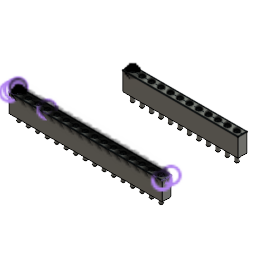
Penguin gameboy (Autodesk Fusion 360 archive; units mm, degrees)
design "Stacking headers 16/12 short v2"
Autodesk Fusion 360 part; units mm, degrees
note: some values were not read from the file. Chosen so that the rebuilt part matches the saved one: which bodies a step acts on.
sketch "Sketch1" plane through (0, 0, 0) normal (0, 1, 0) x (1, 0, 0)
  line L0 (0, 0) -> (41.04, 0)
  line L1 (41.04, 0) -> (41.04, -2.4)
  line L2 (41.04, -2.4) -> (0, -2.4)
  line L3 (0, -2.4) -> (0, 0)
  line L4 (41.04, -1.2) -> (0, -1.2) construction
  circle A0 centre (1.47, -1.2) radius 0.5
  circle A1 centre (4.01, -1.2) radius 0.5
  circle A2 centre (6.55, -1.2) radius 0.5
  circle A3 centre (9.09, -1.2) radius 0.5
  circle A4 centre (11.63, -1.2) radius 0.5
  circle A5 centre (14.17, -1.2) radius 0.5
  circle A6 centre (16.71, -1.2) radius 0.5
  circle A7 centre (19.25, -1.2) radius 0.5
  circle A8 centre (21.79, -1.2) radius 0.5
  circle A9 centre (24.33, -1.2) radius 0.5
  circle A10 centre (26.87, -1.2) radius 0.5
  circle A11 centre (29.41, -1.2) radius 0.5
  circle A12 centre (31.95, -1.2) radius 0.5
  circle A13 centre (34.49, -1.2) radius 0.5
  circle A14 centre (37.03, -1.2) radius 0.5
  circle A15 centre (39.57, -1.2) radius 0.5
  dimension "d1" = 41.04
  dimension "d2" = 2.4
  dimension "d3" = 1
  dimension "d4" = 1.47
  dimension "d11" = -38.1
  dimension "d12" = 0
  constraint horizontal L0
  constraint vertical L1
  constraint horizontal L2
  constraint vertical L3
  constraint coincident L0.start L3.end
  constraint midpoint L1 L4.start
  constraint midpoint L3 L4.end
  constraint coincident L4 A0.centre
  measures "d1" distance of L0.start L0.end
  measures "d2" distance of L0.start L2.end
  measures "d3" diameter of A0
  measures "d4" distance of L3 A0.centre
extrude "Extrude1" add sketch "Sketch1" against normal blind 7 contours A0 | A1 | A2 | A3 | A4 | A5 | A6 | A7 | A8 | A9 | A10 | A11 | A12 | A13 | A14 | A15 makes body 1 at (7.0475, -4.6667, 1.2498) makes body 2 at (16.3609, -4.6667, 0.8421) makes body 3 at (26.5209, -4.6667, 0.8421) makes body 4 at (36.8019, -2.3333, 1.6449) makes body 5 at (34.2619, -2.3333, 1.6449) makes body 6 at (23.9809, -4.6667, 0.8421) makes body 7 at (14.6675, -4.6667, 1.2498) makes body 8 at (4.5075, -4.6667, 1.2498) makes body 9 at (9.5875, -4.6667, 1.2498) makes body 10 at (18.9009, -4.6667, 0.8421) makes body 11 at (29.0609, -4.6667, 0.8421) makes body 12 at (39.3419, -2.3333, 1.6449) makes body 13 at (32.2213, -4.6667, 0.78) makes body 14 at (21.4409, -4.6667, 0.8421) makes body 15 at (12.1275, -4.6667, 1.2498) makes body 16 at (1.9675, -4.6667, 1.2498)
extrude "Extrude2" add sketch "Sketch1" against normal blind 5 bodies 1 2 3 4 5 6 7 8 9 10 11 12 13 14 15 16
fillet "Fillet1" radius 0.5 16 edges at (1.0038, -7, 1.0192) (3.5438, -7, 1.0192) (6.0838, -7, 1.0192) (8.6238, -7, 1.0192) (11.1638, -7, 1.0192) (13.7038, -7, 1.0192) (16.2438, -7, 1.0192) (18.7838, -7, 1.0192) (21.3238, -7, 1.0192) (23.8638, -7, 1.0192) (26.4038, -7, 1.0192) (28.9438, -7, 1.0192) (31.4838, -7, 1.0192) (34.0238, -7, 1.0192) (36.5638, -7, 1.0192) (39.1038, -7, 1.0192) on bodies 1
copy_body "Body->Comp1" bodies 1 removing the originals makes body 17 in component "Component"
sketch "Sketch1 (2)" plane through (0, 0, 0) normal (0, 1, 0) x (1, 0, 0) in component "Component"
  line L0 (10.16, 20.32) -> (41.04, 20.32)
  line L1 (41.04, 20.32) -> (41.04, 17.92)
  line L2 (41.04, 17.92) -> (10.16, 17.92)
  line L3 (10.16, 17.92) -> (10.16, 20.32)
  line L4 (41.04, 0) -> (41.04, -2.4)
  line L5 (41.04, 19.12) -> (10.16, 19.12) construction
  circle A0 centre (11.63, 19.12) radius 0.5
  circle A1 centre (14.17, 19.12) radius 0.5
  circle A2 centre (16.71, 19.12) radius 0.5
  circle A3 centre (19.25, 19.12) radius 0.5
  circle A4 centre (21.79, 19.12) radius 0.5
  circle A5 centre (24.33, 19.12) radius 0.5
  circle A6 centre (26.87, 19.12) radius 0.5
  circle A7 centre (29.41, 19.12) radius 0.5
  circle A8 centre (31.95, 19.12) radius 0.5
  circle A9 centre (34.49, 19.12) radius 0.5
  circle A10 centre (37.03, 19.12) radius 0.5
  circle A11 centre (39.57, 19.12) radius 0.5
  line L6 (0, -2.4) -> (0, 0)
  point P0 (9.09, -1.2)
  point P1 (0, -1.2)
  dimension "d19" = 30.88
  dimension "d20" = 2.4
  dimension "d21" = 1
  dimension "d22" = 1.47
  dimension "d25" = -27.94
  dimension "d26" = 0
  dimension "d27" = 20.32
  constraint horizontal L0
  constraint vertical L1
  constraint horizontal L2
  constraint vertical L3
  constraint midpoint L1 L5.start
  constraint midpoint L3 L5.end
  constraint coincident L5 A0.centre
  constraint collinear L1 L4
  measures "d19" distance of L0.start L0.end
  measures "d20" distance of L0.start L2.end
  measures "d21" diameter of A0
  measures "d22" distance of L3 A0.centre
  measures "d27" vertical distance of A0.centre P0
extrude "Extrude1'" add sketch "Sketch1 (2)" against normal blind 5 separate body makes body 18 in component "Component"
extrude "Extrude2'" add sketch "Sketch1 (2)" against normal blind 7.5 contours A11 bodies 18 in component "Component"
fillet "Fillet1'" radius 0.5 1 edges at (39.1038, -7.5, -19.3008) on bodies 18 in component "Component"
extrude "Extrude3" cut sketch "Sketch1 (2)" against normal blind 2.54 contours A11 bodies 18 in component "Component"
pattern_linear "R-Pattern1" count 12 spacing 2.54 along (-1, 0, 0) of "Extrude2'" in component "Component"
fillet "Fillet2" radius 0.5 11 edges at (36.5638, -7.5, -19.3008) (34.0238, -7.5, -19.3008) (31.4838, -7.5, -19.3008) (28.9438, -7.5, -19.3008) (26.4038, -7.5, -19.3008) (23.8638, -7.5, -19.3008) (21.3238, -7.5, -19.3008) (18.7838, -7.5, -19.3008) (16.2438, -7.5, -19.3008) (13.7038, -7.5, -19.3008) (11.1638, -7.5, -19.3008) on bodies 18 in component "Component"
extrude "Extrude4" cut sketch "Sketch1" against normal blind 2.54 contours A0 | A1 | A2 | A3 | A4 | A5 | A6 | A7 | A8 | A9 | A10 | A11 | A12 | A13 | A14 | A15 bodies 17 in component "Component"
extrude "Extrude5" cut sketch "Sketch1 (2)" against normal blind 4.5 contours A0 | A1 | A2 | A3 | A4 | A5 | A6 | A7 | A8 | A9 | A10 bodies 18 in component "Component"
component "Component" placed x (1, 0, 0) y (0, 1, 0) z (0, 0, 1) at (0, 0, 0)
equation "d1 = ( ( 2.54 * 16 ) * 1 mm ) + 0.4 mm"
equation "d11 = ( -2.54 * 15 ) * 1 mm"
equation "d19 = ( 2.54 * 12 ) * 1 mm + 0.4 mm"
equation "d25 = ( -2.54 * 11 ) * 1 mm"
equation "d38 = ( 2.54 * 11 ) * 1 mm"

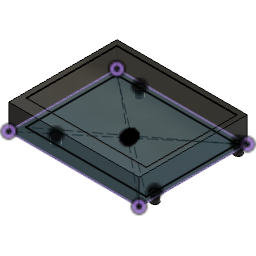
design "SCREEN"
part number: 2025-11-17-10-39-17-028
part number: 2025-11-20-10-21-56-898
Autodesk Fusion 360 part; units mm, degrees
sketch "Sketch1" plane through (0, 0, 0) normal (0, 1, 0) x (1, 0, 0) in component "screen"
  line L0 (38.3, 31.8) -> (-38.3, 31.8)
  line L1 (-38.3, 31.8) -> (-38.3, -31.8)
  line L2 (-38.3, -31.8) -> (38.3, -31.8)
  line L3 (38.3, -31.8) -> (38.3, 31.8)
  line L4 (38.3, 31.8) -> (-38.3, -31.8) construction
  line L5 (-38.3, 31.8) -> (38.3, -31.8) construction
  line L6 (35.34, 28.78) -> (-35.34, 28.78)
  line L7 (-35.34, 28.78) -> (-35.34, -24.58)
  line L8 (-35.34, -24.58) -> (35.34, -24.58)
  line L9 (35.34, -24.58) -> (35.34, 28.78)
  line L10 (35.34, 28.78) -> (-35.34, -24.58) construction
  line L11 (-35.34, 28.78) -> (35.34, -24.58) construction
  point P0 (0, 2.1)
  dimension "d1" = 63.6
  dimension "d2" = 76.6
  dimension "d3" = 70.68
  dimension "d4" = 53.36
  dimension "d7" = 2.96
  dimension "d8" = 3.02
  constraint horizontal L0
  constraint perpendicular L0 L1
  constraint parallel L0 L2
  constraint parallel L1 L3
  constraint coincident L4 origin
  constraint coincident L5 origin
  constraint horizontal L6
  constraint perpendicular L6 L7
  constraint parallel L6 L8
  constraint parallel L7 L9
  constraint coincident L10 P0
  constraint coincident L11 P0
  measures "d1" distance of L0.end L1.end
  measures "d2" distance of L0.start L0.end
  measures "d3" distance of L7.end L8.end
  measures "d4" distance of L6.end L7.end
  measures "d7" distance of L1 L7
  measures "d8" distance of L0 L6
extrude "Extrude1" add sketch "Sketch1" along normal blind 15 in component "screen"
extrude "Extrude2" add sketch "Sketch1" along normal blind 14.5 contours L6 L7 L8 L9 in component "screen"
sketch "Sketch2" plane through (0, 0, 0) normal (0, 1, 0) x (1, 0, 0) in component "screen"
  line L0 (-38.3, -31.8) -> (38.3, -31.8)
  circle A0 centre (35.29, -19.52) radius 2.32
  circle A1 centre (-22.71, -19.52) radius 2.32
  circle A2 centre (35.29, 29.48) radius 2.32
  circle A3 centre (-22.71, 29.48) radius 2.32
  line L1 (38.3, -31.8) -> (38.3, 31.8)
  line L2 (-38.3, 31.8) -> (-38.3, -31.8)
  line L3 (38.3, 31.8) -> (-38.3, 31.8)
  dimension "d17" = 12.28
  dimension "d20" = -58
  dimension "d21" = 49
  dimension "d24" = 15.59
  constraint tangent A2 L3
  measures "d17" distance of L0 A0.centre
  measures "d24" distance of A3.centre L2
extrude "Extrude3" add sketch "Sketch2" against normal blind 5 contours A2 | A3 | A0 | A1 in component "screen"
component "screen" placed x (1, 0, 0) y (0, 1, 0) z (0, 0, 1) at (0, 0, 0)
equation "d7 = ( 5.92 / 2 ) * 1 mm"

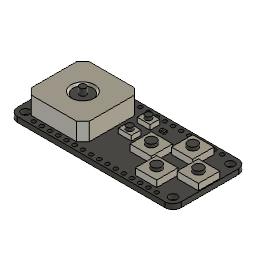
design "3632 Joy FeatherWing (bad)"
Autodesk Fusion 360 part; units mm, degrees
sketch "PCB" plane through (0, 0, 0) normal (0, 0, 1) x (1, 0, 0)
  arc A0 (50.8, 20.32) -> (48.26, 22.86) centre (48.26, 20.32) ccw
  arc A1 (48.26, 0) -> (50.8, 2.54) centre (48.26, 2.54) ccw
  line L0 (2.54, 22.86) -> (48.26, 22.86)
  line L1 (0, 20.32) -> (0, 2.54)
  circle A2 centre (5.43, 5.43) radius 0.8
  arc A3 (0, 2.54) -> (2.54, 0) centre (2.54, 2.54) ccw
  line L2 (48.26, 0) -> (2.54, 0)
  arc A4 (0, 2.54) -> (2.54, 0) centre (2.54, 2.54) ccw
  circle A5 centre (17.43, 17.43) radius 0.8
  arc A6 (50.8, 20.32) -> (48.26, 22.86) centre (48.26, 20.32) ccw
  line L3 (50.8, 2.54) -> (50.8, 20.32)
  arc A7 (48.26, 0) -> (50.8, 2.54) centre (48.26, 2.54) ccw
  line L4 (50.8, 20.32) -> (50.8, 2.54)
  line L5 (2.54, 0) -> (48.26, 0)
  arc A8 (2.54, 22.86) -> (0, 20.32) centre (2.54, 20.32) ccw
  arc A9 (2.54, 22.86) -> (0, 20.32) centre (2.54, 20.32) ccw
  line L6 (48.26, 22.86) -> (2.54, 22.86)
  line L7 (0, 2.54) -> (0, 20.32)
  circle A10 centre (2.54, 2.54) radius 1.27
  circle A11 centre (2.54, 20.32) radius 1.27
  circle A12 centre (2.43, 13.43) radius 0.635
  circle A13 centre (2.43, 11.43) radius 0.635
  circle A14 centre (2.43, 9.43) radius 0.635
  circle A15 centre (9.43, 20.43) radius 0.635
  circle A16 centre (11.43, 20.43) radius 0.635
  circle A17 centre (13.43, 20.43) radius 0.635
  circle A18 centre (48.26, 20.32) radius 1.27
  circle A19 centre (48.26, 2.54) radius 1.27
  circle A20 centre (6.35, 1.27) radius 0.635
  circle A21 centre (8.89, 1.27) radius 0.635
  circle A22 centre (11.43, 1.27) radius 0.635
  circle A23 centre (13.97, 1.27) radius 0.635
  circle A24 centre (16.51, 1.27) radius 0.635
  circle A25 centre (19.05, 1.27) radius 0.635
  circle A26 centre (21.59, 1.27) radius 0.635
  circle A27 centre (24.13, 1.27) radius 0.635
  circle A28 centre (26.67, 1.27) radius 0.635
  circle A29 centre (29.21, 1.27) radius 0.635
  circle A30 centre (31.75, 1.27) radius 0.635
  circle A31 centre (34.29, 1.27) radius 0.635
  circle A32 centre (36.83, 1.27) radius 0.635
  circle A33 centre (39.37, 1.27) radius 0.635
  circle A34 centre (41.91, 1.27) radius 0.635
  circle A35 centre (44.45, 1.27) radius 0.635
  circle A36 centre (16.51, 21.59) radius 0.635
  circle A37 centre (19.05, 21.59) radius 0.635
  circle A38 centre (21.59, 21.59) radius 0.635
  circle A39 centre (24.13, 21.59) radius 0.635
  circle A40 centre (26.67, 21.59) radius 0.635
  circle A41 centre (29.21, 21.59) radius 0.635
  circle A42 centre (31.75, 21.59) radius 0.635
  circle A43 centre (34.29, 21.59) radius 0.635
  circle A44 centre (36.83, 21.59) radius 0.635
  circle A45 centre (39.37, 21.59) radius 0.635
  circle A46 centre (41.91, 21.59) radius 0.635
  circle A47 centre (44.45, 21.59) radius 0.635
  dimension "d1" = 2.54
  dimension "d2" = 2.54
  dimension "d3" = 1.27
  dimension "d4" = 1.27
  dimension "d5" = 1.27
  dimension "d6" = 1.27
  dimension "d7" = 1.27
  dimension "d8" = 1.27
  dimension "d9" = 2.54
  dimension "d10" = 2.54
  dimension "d11" = 1.27
  dimension "d14" = 2.54
  dimension "d15" = 0
  dimension "d16" = 1.27
  dimension "d19" = 2.54
  dimension "d20" = 0
  constraint concentric A3 A10
  constraint concentric A8 A11
  constraint concentric A0 A18
  constraint concentric A1 A19
  measures "d1" diameter of A10
  measures "d2" diameter of A11
  measures "d3" diameter of A12
  measures "d4" diameter of A13
  measures "d5" diameter of A14
  measures "d6" diameter of A15
  measures "d7" diameter of A16
  measures "d8" diameter of A17
  measures "d9" diameter of A18
  measures "d10" diameter of A19
  measures "d11" diameter of A20
  measures "d16" diameter of A36
extrude "Extrude1" add sketch "PCB" along normal blind 1.6 makes body 1
sketch "thumbstick" plane through (0, 0, 1.6) normal (0, 0, 1) x (-1, 0, 0)
  circle A0 centre (-31.75, -21.59) radius 0.635
  circle A1 centre (-8.89, -1.27) radius 0.635
  circle A2 centre (-19.05, -1.27) radius 0.635
  circle A3 centre (-16.51, -1.27) radius 0.635
  circle A4 centre (-41.91, -21.59) radius 0.635
  circle A5 centre (-2.54, -2.54) radius 1.27 construction
  circle A6 centre (-39.37, -21.59) radius 0.635
  circle A7 centre (-24.13, -1.27) radius 0.635
  circle A8 centre (-13.97, -1.27) radius 0.635
  circle A9 centre (-36.83, -21.59) radius 0.635
  circle A10 centre (-48.26, -2.54) radius 1.27
  circle A11 centre (-6.35, -1.27) radius 0.635
  circle A12 centre (-11.43, -1.27) radius 0.635
  circle A13 centre (-2.43, -13.43) radius 0.635 construction
  circle A14 centre (-2.54, -20.32) radius 1.27 construction
  circle A15 centre (-44.45, -21.59) radius 0.635
  circle A16 centre (-17.43, -17.43) radius 0.8 construction
  circle A17 centre (-11.43, -20.43) radius 0.635 construction
  circle A18 centre (-9.43, -20.43) radius 0.635 construction
  circle A19 centre (-34.29, -1.27) radius 0.635
  circle A20 centre (-24.13, -21.59) radius 0.635
  circle A21 centre (-2.43, -9.43) radius 0.635 construction
  circle A22 centre (-31.75, -1.27) radius 0.635
  circle A23 centre (-2.43, -11.43) radius 0.635 construction
  circle A24 centre (-21.59, -1.27) radius 0.635
  circle A25 centre (-16.51, -21.59) radius 0.635
  circle A26 centre (-48.26, -20.32) radius 1.27
  circle A27 centre (-21.59, -21.59) radius 0.635
  circle A28 centre (-39.37, -1.27) radius 0.635
  circle A29 centre (-29.21, -1.27) radius 0.635
  circle A30 centre (-41.91, -1.27) radius 0.635
  circle A31 centre (-13.43, -20.43) radius 0.635 construction
  circle A32 centre (-34.29, -21.59) radius 0.635
  circle A33 centre (-26.67, -1.27) radius 0.635
  circle A34 centre (-26.67, -21.59) radius 0.635
  circle A35 centre (-19.05, -21.59) radius 0.635
  circle A36 centre (-44.45, -1.27) radius 0.635
  circle A37 centre (-36.83, -1.27) radius 0.635
  circle A38 centre (-29.21, -21.59) radius 0.635
  circle A39 centre (-5.43, -5.43) radius 0.8 construction
  line L0 (-2.54, 0) -> (-48.26, 0)
  arc A40 (-48.26, 0) -> (-50.8, -2.54) centre (-48.26, -2.54) ccw
  line L1 (-50.8, -2.54) -> (-50.8, -20.32)
  arc A41 (-50.8, -20.32) -> (-48.26, -22.86) centre (-48.26, -20.32) ccw
  line L2 (-48.26, -22.86) -> (-2.54, -22.86)
  arc A42 (-2.54, -22.86) -> (0, -20.32) centre (-2.54, -20.32) ccw
  line L3 (0, -20.32) -> (0, -2.54)
  arc A43 (0, -2.54) -> (-2.54, 0) centre (-2.54, -2.54) ccw
  line L4 (-20.43, -2.43) -> (-2.43, -2.43)
  line L5 (-2.43, -2.43) -> (-2.43, -20.43)
  line L6 (-2.43, -20.43) -> (-20.43, -20.43)
  line L7 (-20.43, -20.43) -> (-20.43, -2.43)
  line L8 (-20.43, -2.43) -> (-2.43, -20.43) construction
  line L9 (-2.43, -2.43) -> (-20.43, -20.43) construction
  point P0 (-11.43, -11.43)
  dimension "d23" = 18
  dimension "d24" = 18
  dimension "d25" = 11.43
  dimension "d26" = 11.43
  constraint perpendicular L4 L5
  constraint parallel L4 L6
  constraint parallel L5 L7
  constraint horizontal L4
  constraint coincident L8 P0
  constraint coincident L9 P0
  measures "d23" distance of L5.end L6.end
  measures "d24" distance of L4.end L5.end
  measures "d25" distance of L3 P0
  measures "d26" distance of L0 P0
extrude "Extrude2" add sketch "thumbstick" along normal blind 5.5 separate body contours L4 L5 L6 L7 makes body 2
chamfer "Chamfer1" distance 2 angle 45 4 edges at (2.43, 2.43, 4.35) (2.43, 20.43, 4.35) (20.43, 20.43, 4.35) (20.43, 2.43, 4.35) on bodies 2
sketch "stem" plane through (0, 0, 7.1) normal (0, 0, 1) x (-1, 0, 0)
  line L0 (-18.43, -2.43) -> (-20.43, -4.43)
  line L1 (-20.43, -4.43) -> (-20.43, -18.43)
  line L2 (-20.43, -18.43) -> (-18.43, -20.43)
  line L3 (-18.43, -20.43) -> (-4.43, -20.43)
  line L4 (-4.43, -20.43) -> (-2.43, -18.43)
  line L5 (-2.43, -18.43) -> (-2.43, -4.43)
  line L6 (-2.43, -4.43) -> (-4.43, -2.43)
  line L7 (-4.43, -2.43) -> (-18.43, -2.43)
  line L8 (-11.43, -20.43) -> (-11.43, -2.43) construction
  line L9 (-2.43, -11.43) -> (-20.43, -11.43) construction
  circle A0 centre (-11.43, -11.43) radius 3
  circle A1 centre (-11.43, -11.43) radius 1
  dimension "d30" = 6
  dimension "d34" = 2
  constraint midpoint L3 L8.start
  constraint midpoint L7 L8.end
  constraint midpoint L5 L9.start
  constraint midpoint L1 L9.end
  constraint midpoint L9 A0.centre
  constraint concentric A0 A1
  measures "d30" diameter of A0
  measures "d34" diameter of A1
extrude "Extrude3" cut sketch "stem" against normal blind 0.6 contours A0 | A1 bodies 2
chamfer "Chamfer2" distance 0.6 angle 45 1 edges at (14.227, 10.3452, 7.1) on bodies 2
extrude "Extrude4" add sketch "stem" along normal blind 2 from surface at -0.6 contours A1 bodies 2
sketch "select reset" plane through (0, 0, 1.6) normal (0, 0, 1) x (-1, 0, 0)
  circle A0 centre (-31.75, -21.59) radius 0.635
  circle A1 centre (-8.89, -1.27) radius 0.635
  circle A2 centre (-19.05, -1.27) radius 0.635
  circle A3 centre (-16.51, -1.27) radius 0.635
  circle A4 centre (-41.91, -21.59) radius 0.635
  circle A5 centre (-2.54, -2.54) radius 1.27
  circle A6 centre (-39.37, -21.59) radius 0.635
  circle A7 centre (-24.13, -1.27) radius 0.635
  circle A8 centre (-13.97, -1.27) radius 0.635
  circle A9 centre (-36.83, -21.59) radius 0.635
  circle A10 centre (-48.26, -2.54) radius 1.27
  circle A11 centre (-6.35, -1.27) radius 0.635
  circle A12 centre (-11.43, -1.27) radius 0.635
  circle A13 centre (-2.43, -13.43) radius 0.635
  circle A14 centre (-2.54, -20.32) radius 1.27
  circle A15 centre (-44.45, -21.59) radius 0.635
  circle A16 centre (-17.43, -17.43) radius 0.8
  circle A17 centre (-11.43, -20.43) radius 0.635
  circle A18 centre (-9.43, -20.43) radius 0.635
  circle A19 centre (-34.29, -1.27) radius 0.635
  circle A20 centre (-24.13, -21.59) radius 0.635
  circle A21 centre (-2.43, -9.43) radius 0.635
  circle A22 centre (-31.75, -1.27) radius 0.635
  circle A23 centre (-2.43, -11.43) radius 0.635
  circle A24 centre (-21.59, -1.27) radius 0.635
  circle A25 centre (-16.51, -21.59) radius 0.635
  circle A26 centre (-48.26, -20.32) radius 1.27
  circle A27 centre (-21.59, -21.59) radius 0.635
  circle A28 centre (-39.37, -1.27) radius 0.635
  circle A29 centre (-29.21, -1.27) radius 0.635
  circle A30 centre (-41.91, -1.27) radius 0.635
  circle A31 centre (-13.43, -20.43) radius 0.635
  circle A32 centre (-34.29, -21.59) radius 0.635
  circle A33 centre (-26.67, -1.27) radius 0.635
  circle A34 centre (-26.67, -21.59) radius 0.635
  circle A35 centre (-19.05, -21.59) radius 0.635
  circle A36 centre (-44.45, -1.27) radius 0.635
  circle A37 centre (-36.83, -1.27) radius 0.635
  circle A38 centre (-29.21, -21.59) radius 0.635
  circle A39 centre (-5.43, -5.43) radius 0.8
  line L0 (-2.54, 0) -> (-48.26, 0)
  arc A40 (-48.26, 0) -> (-50.8, -2.54) centre (-48.26, -2.54) ccw
  line L1 (-50.8, -2.54) -> (-50.8, -20.32)
  arc A41 (-50.8, -20.32) -> (-48.26, -22.86) centre (-48.26, -20.32) ccw
  line L2 (-48.26, -22.86) -> (-2.54, -22.86)
  arc A42 (-2.54, -22.86) -> (0, -20.32) centre (-2.54, -20.32) ccw
  line L3 (0, -20.32) -> (0, -2.54)
  arc A43 (0, -2.54) -> (-2.54, 0) centre (-2.54, -2.54) ccw
  line L4 (-26.765, -16.915) -> (-22.765, -16.915)
  line L5 (-22.765, -16.915) -> (-22.765, -19.915)
  line L6 (-22.765, -19.915) -> (-26.765, -19.915)
  line L7 (-26.765, -19.915) -> (-26.765, -16.915)
  line L8 (-26.765, -16.915) -> (-22.765, -19.915) construction
  line L9 (-22.765, -16.915) -> (-26.765, -19.915) construction
  line L10 (-26.765, -11.073) -> (-22.765, -11.073)
  line L11 (-22.765, -11.073) -> (-22.765, -14.073)
  line L12 (-22.765, -14.073) -> (-26.765, -14.073)
  line L13 (-26.765, -14.073) -> (-26.765, -11.073)
  line L14 (-26.765, -11.073) -> (-22.765, -14.073) construction
  line L15 (-22.765, -11.073) -> (-26.765, -14.073) construction
  circle A44 centre (-24.765, -18.415) radius 1
  circle A45 centre (-24.765, -12.573) radius 1
  point P0 (-24.765, -18.415)
  point P1 (-24.765, -12.573)
  dimension "d38" = 4
  dimension "d39" = 3
  dimension "d40" = 24.765
  dimension "d41" = 18.415
  dimension "d42" = 4
  dimension "d43" = 3
  dimension "d44" = 24.765
  dimension "d45" = 12.573
  dimension "d48" = 2
  dimension "d49" = 2
  constraint perpendicular L4 L5
  constraint parallel L4 L6
  constraint parallel L5 L7
  constraint horizontal L4
  constraint coincident L8 P0
  constraint coincident L9 P0
  constraint perpendicular L10 L11
  constraint parallel L10 L12
  constraint parallel L11 L13
  constraint horizontal L10
  constraint coincident L14 P1
  constraint coincident L15 P1
  constraint coincident P0 A44.centre
  constraint coincident P1 A45.centre
  measures "d38" distance of L5.end L6.end
  measures "d39" distance of L4.end L5.end
  measures "d40" distance of L3 P0
  measures "d41" distance of L0 P0
  measures "d42" distance of L11.end L12.end
  measures "d43" distance of L10.end L11.end
  measures "d44" distance of L3 P1
  measures "d45" distance of L0 P1
  measures "d48" diameter of A44
  measures "d49" diameter of A45
extrude "Extrude5" add sketch "select reset" along normal blind 1.5 separate body contours L4 L5 L6 L7 | L10 L11 L12 L13 | A44 | A45 makes body 3 at (25.4317, 17.915, 1.6) makes body 4 at (25.4317, 12.073, 1.6)
extrude "Extrude6" add sketch "select reset" along normal blind 1 from surface at 1.5 contours A44 | A45 bodies 3 4
sketch "action buttons" plane through (0, 0, 1.6) normal (0, 0, 1) x (-1, 0, 0)
  circle A0 centre (-31.75, -21.59) radius 0.635
  circle A1 centre (-8.89, -1.27) radius 0.635
  circle A2 centre (-19.05, -1.27) radius 0.635
  circle A3 centre (-16.51, -1.27) radius 0.635
  circle A4 centre (-41.91, -21.59) radius 0.635
  circle A5 centre (-2.54, -2.54) radius 1.27
  circle A6 centre (-39.37, -21.59) radius 0.635
  circle A7 centre (-24.13, -1.27) radius 0.635
  circle A8 centre (-13.97, -1.27) radius 0.635
  circle A9 centre (-36.83, -21.59) radius 0.635
  circle A10 centre (-48.26, -2.54) radius 1.27
  circle A11 centre (-6.35, -1.27) radius 0.635
  circle A12 centre (-11.43, -1.27) radius 0.635
  circle A13 centre (-2.43, -13.43) radius 0.635
  circle A14 centre (-2.54, -20.32) radius 1.27
  circle A15 centre (-44.45, -21.59) radius 0.635
  circle A16 centre (-17.43, -17.43) radius 0.8
  circle A17 centre (-11.43, -20.43) radius 0.635
  circle A18 centre (-9.43, -20.43) radius 0.635
  circle A19 centre (-34.29, -1.27) radius 0.635
  circle A20 centre (-24.13, -21.59) radius 0.635
  circle A21 centre (-2.43, -9.43) radius 0.635
  circle A22 centre (-31.75, -1.27) radius 0.635
  circle A23 centre (-2.43, -11.43) radius 0.635
  circle A24 centre (-21.59, -1.27) radius 0.635
  circle A25 centre (-16.51, -21.59) radius 0.635
  circle A26 centre (-48.26, -20.32) radius 1.27
  circle A27 centre (-21.59, -21.59) radius 0.635
  circle A28 centre (-39.37, -1.27) radius 0.635
  circle A29 centre (-29.21, -1.27) radius 0.635
  circle A30 centre (-41.91, -1.27) radius 0.635
  circle A31 centre (-13.43, -20.43) radius 0.635
  circle A32 centre (-34.29, -21.59) radius 0.635
  circle A33 centre (-26.67, -1.27) radius 0.635
  circle A34 centre (-26.67, -21.59) radius 0.635
  circle A35 centre (-19.05, -21.59) radius 0.635
  circle A36 centre (-44.45, -1.27) radius 0.635
  circle A37 centre (-36.83, -1.27) radius 0.635
  circle A38 centre (-29.21, -21.59) radius 0.635
  circle A39 centre (-5.43, -5.43) radius 0.8
  line L0 (-2.54, 0) -> (-48.26, 0)
  arc A40 (-48.26, 0) -> (-50.8, -2.54) centre (-48.26, -2.54) ccw
  line L1 (-50.8, -2.54) -> (-50.8, -20.32)
  arc A41 (-50.8, -20.32) -> (-48.26, -22.86) centre (-48.26, -20.32) ccw
  line L2 (-48.26, -22.86) -> (-2.54, -22.86)
  arc A42 (-2.54, -22.86) -> (0, -20.32) centre (-2.54, -20.32) ccw
  line L3 (0, -20.32) -> (0, -2.54)
  arc A43 (0, -2.54) -> (-2.54, 0) centre (-2.54, -2.54) ccw
  line L4 (-35.939, -8.13) -> (-29.339, -8.13)
  line L5 (-29.339, -8.13) -> (-29.339, -14.73)
  line L6 (-29.339, -14.73) -> (-35.939, -14.73)
  line L7 (-35.939, -14.73) -> (-35.939, -8.13)
  line L8 (-35.939, -8.13) -> (-29.339, -14.73) construction
  line L9 (-29.339, -8.13) -> (-35.939, -14.73) construction
  line L10 (-43.178, -13.718) -> (-36.578, -13.718)
  line L11 (-36.578, -13.718) -> (-36.578, -20.318)
  line L12 (-36.578, -20.318) -> (-43.178, -20.318)
  line L13 (-43.178, -20.318) -> (-43.178, -13.718)
  line L14 (-43.178, -13.718) -> (-36.578, -20.318) construction
  line L15 (-36.578, -13.718) -> (-43.178, -20.318) construction
  line L16 (-43.178, -2.542) -> (-36.578, -2.542)
  line L17 (-36.578, -2.542) -> (-36.578, -9.142)
  line L18 (-36.578, -9.142) -> (-43.178, -9.142)
  line L19 (-43.178, -9.142) -> (-43.178, -2.542)
  line L20 (-43.178, -2.542) -> (-36.578, -9.142) construction
  line L21 (-36.578, -2.542) -> (-43.178, -9.142) construction
  line L22 (-50.544, -8.13) -> (-43.944, -8.13)
  line L23 (-43.944, -8.13) -> (-43.944, -14.73)
  line L24 (-43.944, -14.73) -> (-50.544, -14.73)
  line L25 (-50.544, -14.73) -> (-50.544, -8.13)
  line L26 (-50.544, -8.13) -> (-43.944, -14.73) construction
  line L27 (-43.944, -8.13) -> (-50.544, -14.73) construction
  circle A44 centre (-32.639, -11.43) radius 1.5
  circle A45 centre (-39.878, -17.018) radius 1.5
  circle A46 centre (-39.878, -5.842) radius 1.5
  circle A47 centre (-47.244, -11.43) radius 1.5
  point P0 (-32.639, -11.43)
  point P1 (-39.878, -17.018)
  point P2 (-39.878, -5.842)
  point P3 (-47.244, -11.43)
  dimension "d53" = 6.6
  dimension "d54" = 6.6
  dimension "d55" = 32.639
  dimension "d56" = 11.43
  dimension "d57" = 6.6
  dimension "d58" = 6.6
  dimension "d59" = 39.878
  dimension "d60" = 17.018
  dimension "d61" = 6.6
  dimension "d62" = 6.6
  dimension "d63" = 39.878
  dimension "d64" = 5.842
  dimension "d65" = 6.6
  dimension "d66" = 6.6
  dimension "d67" = 11.43
  dimension "d68" = 47.244
  dimension "d69" = 3
  dimension "d70" = 3
  dimension "d71" = 3
  dimension "d72" = 3
  constraint perpendicular L4 L5
  constraint parallel L4 L6
  constraint parallel L5 L7
  constraint horizontal L4
  constraint coincident L8 P0
  constraint coincident L9 P0
  constraint perpendicular L10 L11
  constraint parallel L10 L12
  constraint parallel L11 L13
  constraint horizontal L10
  constraint coincident L14 P1
  constraint coincident L15 P1
  constraint perpendicular L16 L17
  constraint parallel L16 L18
  constraint parallel L17 L19
  constraint horizontal L16
  constraint coincident L20 P2
  constraint coincident L21 P2
  constraint perpendicular L22 L23
  constraint parallel L22 L24
  constraint parallel L23 L25
  constraint horizontal L22
  constraint coincident L26 P3
  constraint coincident L27 P3
  constraint coincident P0 A44.centre
  constraint coincident P1 A45.centre
  constraint coincident P2 A46.centre
  constraint coincident P3 A47.centre
  measures "d53" distance of L5.end L6.end
  measures "d54" distance of L4.end L5.end
  measures "d55" distance of L3 P0
  measures "d56" distance of L0 P0
  measures "d57" distance of L11.end L12.end
  measures "d58" distance of L10.end L11.end
  measures "d59" distance of L3 P1
  measures "d60" distance of L0 P1
  measures "d61" distance of L17.end L18.end
  measures "d62" distance of L16.end L17.end
  measures "d63" distance of L3 P2
  measures "d64" distance of L0 P2
  measures "d65" distance of L22.end L23.end
  measures "d66" distance of L23.end L24.end
  measures "d67" distance of L0 P3
  measures "d68" distance of L3 P3
  measures "d69" diameter of A44
  measures "d70" diameter of A45
  measures "d71" diameter of A46
  measures "d72" diameter of A47
extrude "Extrude7" add sketch "action buttons" along normal blind 2 separate body contours L4 L5 L6 L7 | L10 L11 L12 L13 | L16 L17 L18 L19 | L22 L23 L24 L25 | A44 | A45 | A46 | A47 makes body 5 at (33.739, 10.33, 1.6) makes body 6 at (40.978, 6.942, 1.6) makes body 7 at (40.978, 18.118, 1.6) makes body 8 at (48.344, 10.33, 1.6)
extrude "Extrude8" add sketch "action buttons" along normal blind 1 from surface at 2 contours A44 | A45 | A46 | A47 bodies 5 6 7 8
sketch "Act LED" plane through (0, 0, 1.6) normal (0, 0, 1) x (-1, 0, 0)
  circle A0 centre (-31.75, -21.59) radius 0.635
  circle A1 centre (-8.89, -1.27) radius 0.635
  circle A2 centre (-19.05, -1.27) radius 0.635
  circle A3 centre (-16.51, -1.27) radius 0.635
  circle A4 centre (-41.91, -21.59) radius 0.635
  circle A5 centre (-2.54, -2.54) radius 1.27
  circle A6 centre (-39.37, -21.59) radius 0.635
  circle A7 centre (-24.13, -1.27) radius 0.635
  circle A8 centre (-13.97, -1.27) radius 0.635
  circle A9 centre (-36.83, -21.59) radius 0.635
  circle A10 centre (-48.26, -2.54) radius 1.27
  circle A11 centre (-6.35, -1.27) radius 0.635
  circle A12 centre (-11.43, -1.27) radius 0.635
  circle A13 centre (-2.43, -13.43) radius 0.635
  circle A14 centre (-2.54, -20.32) radius 1.27
  circle A15 centre (-44.45, -21.59) radius 0.635
  circle A16 centre (-17.43, -17.43) radius 0.8
  circle A17 centre (-11.43, -20.43) radius 0.635
  circle A18 centre (-9.43, -20.43) radius 0.635
  circle A19 centre (-34.29, -1.27) radius 0.635
  circle A20 centre (-24.13, -21.59) radius 0.635
  circle A21 centre (-2.43, -9.43) radius 0.635
  circle A22 centre (-31.75, -1.27) radius 0.635
  circle A23 centre (-2.43, -11.43) radius 0.635
  circle A24 centre (-21.59, -1.27) radius 0.635
  circle A25 centre (-16.51, -21.59) radius 0.635
  circle A26 centre (-48.26, -20.32) radius 1.27
  circle A27 centre (-21.59, -21.59) radius 0.635
  circle A28 centre (-39.37, -1.27) radius 0.635
  circle A29 centre (-29.21, -1.27) radius 0.635
  circle A30 centre (-41.91, -1.27) radius 0.635
  circle A31 centre (-13.43, -20.43) radius 0.635
  circle A32 centre (-34.29, -21.59) radius 0.635
  circle A33 centre (-26.67, -1.27) radius 0.635
  circle A34 centre (-26.67, -21.59) radius 0.635
  circle A35 centre (-19.05, -21.59) radius 0.635
  circle A36 centre (-44.45, -1.27) radius 0.635
  circle A37 centre (-36.83, -1.27) radius 0.635
  circle A38 centre (-29.21, -21.59) radius 0.635
  circle A39 centre (-5.43, -5.43) radius 0.8
  line L0 (-2.54, 0) -> (-48.26, 0)
  arc A40 (-48.26, 0) -> (-50.8, -2.54) centre (-48.26, -2.54) ccw
  line L1 (-50.8, -2.54) -> (-50.8, -20.32)
  arc A41 (-50.8, -20.32) -> (-48.26, -22.86) centre (-48.26, -20.32) ccw
  line L2 (-48.26, -22.86) -> (-2.54, -22.86)
  arc A42 (-2.54, -22.86) -> (0, -20.32) centre (-2.54, -20.32) ccw
  line L3 (0, -20.32) -> (0, -2.54)
  arc A43 (0, -2.54) -> (-2.54, 0) centre (-2.54, -2.54) ccw
  line L4 (-30.087, -17.915) -> (-28.587, -17.915)
  line L5 (-28.587, -17.915) -> (-28.587, -18.915)
  line L6 (-28.587, -18.915) -> (-30.087, -18.915)
  line L7 (-30.087, -18.915) -> (-30.087, -17.915)
  line L8 (-30.087, -17.915) -> (-28.587, -18.915) construction
  line L9 (-28.587, -17.915) -> (-30.087, -18.915) construction
  point P0 (-29.337, -18.415)
  dimension "d78" = 1
  dimension "d79" = 1.5
  dimension "d80" = 29.337
  dimension "d81" = 18.415
  constraint perpendicular L4 L5
  constraint parallel L4 L6
  constraint parallel L5 L7
  constraint horizontal L4
  constraint coincident L8 P0
  constraint coincident L9 P0
  measures "d78" distance of L4.end L5.end
  measures "d79" distance of L5.end L6.end
  measures "d80" distance of L3 P0
  measures "d81" distance of L0 P0
extrude "Extrude9" add sketch "Act LED" along normal blind 0.5 separate body contours L4 L5 L6 L7 makes body 9
named bodies: "pcb", "thumbstick", "select", "reset", "LED"

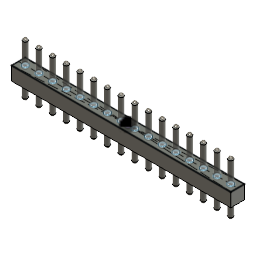
design "Standard Pins 16"
Autodesk Fusion 360 part; units mm, degrees
sketch "Sketch1" plane through (0, 0, 0) normal (0, 1, 0) x (1, 0, 0) in component "Standard 16 Pins"
  line L0 (20.32, 1.27) -> (-20.32, 1.27)
  line L1 (-20.32, 1.27) -> (-20.32, -1.27)
  line L2 (-20.32, -1.27) -> (20.32, -1.27)
  line L3 (20.32, -1.27) -> (20.32, 1.27)
  line L4 (20.32, 1.27) -> (-20.32, -1.27) construction
  line L5 (-20.32, 1.27) -> (20.32, -1.27) construction
  circle A0 centre (-19.05, 0) radius 0.45
  line L6 (-20.32, 0) -> (20.32, 0) construction
  circle A1 centre (-16.51, 0) radius 0.45
  circle A2 centre (-13.97, 0) radius 0.45
  circle A3 centre (-11.43, 0) radius 0.45
  circle A4 centre (-8.89, 0) radius 0.45
  circle A5 centre (-6.35, 0) radius 0.45
  circle A6 centre (-3.81, 0) radius 0.45
  circle A7 centre (-1.27, 0) radius 0.45
  circle A8 centre (1.27, 0) radius 0.45
  circle A9 centre (3.81, 0) radius 0.45
  circle A10 centre (6.35, 0) radius 0.45
  circle A11 centre (8.89, 0) radius 0.45
  circle A12 centre (11.43, 0) radius 0.45
  circle A13 centre (13.97, 0) radius 0.45
  circle A14 centre (16.51, 0) radius 0.45
  circle A15 centre (19.05, 0) radius 0.45
  dimension "d1" = 40.64
  dimension "d2" = 2.54
  dimension "d3" = 0.9
  dimension "d4" = 1.27
  dimension "d7" = 38.1
  dimension "d8" = 0
  constraint horizontal L0
  constraint perpendicular L0 L1
  constraint parallel L0 L2
  constraint parallel L1 L3
  constraint coincident L4 origin
  constraint coincident L5 origin
  constraint midpoint L1 L6.start
  constraint midpoint L3 L6.end
  measures "d1" distance of L1.end L2.end
  measures "d2" distance of L0.end L1.end
  measures "d3" diameter of A0
  measures "d4" distance of L1 A0.centre
extrude "Extrude1" add sketch "Sketch1" along normal blind 4.5 and the other way blind 5.54 contours A0 | A1 | A2 | A3 | A4 | A5 | A6 | A7 | A8 | A9 | A10 | A11 | A12 | A13 | A14 | A15 makes body 1 at (14.4194, -3.6933, 0.0224) makes body 2 at (4.2594, -3.6933, 0.0224) makes body 3 at (-5.9006, -3.6933, 0.0224) makes body 4 at (-16.7153, -3.6933, -0.4004) makes body 5 at (-13.8481, -3.6933, -0.4332) makes body 6 at (-3.3606, -3.6933, 0.0224) makes body 7 at (6.7994, -3.6933, 0.0224) makes body 8 at (16.1958, -3.6933, -0.3221) makes body 9 at (11.8794, -3.6933, 0.0224) makes body 10 at (1.7194, -3.6933, 0.0224) makes body 11 at (-8.4406, -3.6933, 0.0224) makes body 12 at (-19.3642, -3.6933, -0.3221) makes body 13 at (-10.9806, -3.6933, 0.0224) makes body 14 at (-0.8206, -3.6933, 0.0224) makes body 15 at (9.0119, -3.6933, -0.4332) makes body 16 at (18.8447, -3.6933, -0.4004) in component "Standard 16 Pins"
extrude "Extrude2" add sketch "Sketch1" against normal blind 2.54 bodies 1 2 3 4 5 6 7 8 9 10 11 12 13 14 15 16 in component "Standard 16 Pins"
fillet "Fillet1" radius 0.45 32 edges at (18.6305, 4.5, 0.1627) (16.0905, 4.5, 0.1627) (13.5505, 4.5, 0.1627) (11.0105, 4.5, 0.1627) (8.4705, 4.5, 0.1627) (5.9305, 4.5, 0.1627) (3.3905, 4.5, 0.1627) (0.8505, 4.5, 0.1627) (-1.6895, 4.5, 0.1627) (-4.2295, 4.5, 0.1627) (-6.7695, 4.5, 0.1627) (-9.3095, 4.5, 0.1627) (-11.8495, 4.5, 0.1627) (-14.3895, 4.5, 0.1627) (-16.9295, 4.5, 0.1627) (-19.4695, 4.5, 0.1627) (18.6305, -5.54, -0.1627) (16.0905, -5.54, -0.1627) (13.5505, -5.54, -0.1627) (11.0105, -5.54, -0.1627) (8.4705, -5.54, -0.1627) (5.9305, -5.54, -0.1627) (3.3905, -5.54, -0.1627) (0.8505, -5.54, -0.1627) (-1.6895, -5.54, -0.1627) (-4.2295, -5.54, -0.1627) (-6.7695, -5.54, -0.1627) (-9.3095, -5.54, -0.1627) (-11.8495, -5.54, -0.1627) (-14.3895, -5.54, -0.1627) (-16.9295, -5.54, -0.1627) (-19.4695, -5.54, -0.1627) on bodies 1 in component "Standard 16 Pins"
component "Standard 16 Pins" placed x (1, 0, 0) y (0, 1, 0) z (0, 0, 1) at (0, 0, 0)
equation "d1 = ( 16 * 2.54 ) * 1 mm"
equation "d4 = ( 2.54 / 2 ) * 1 mm"
equation "d7 = ( 2.54 * 15 ) * 1 mm"
